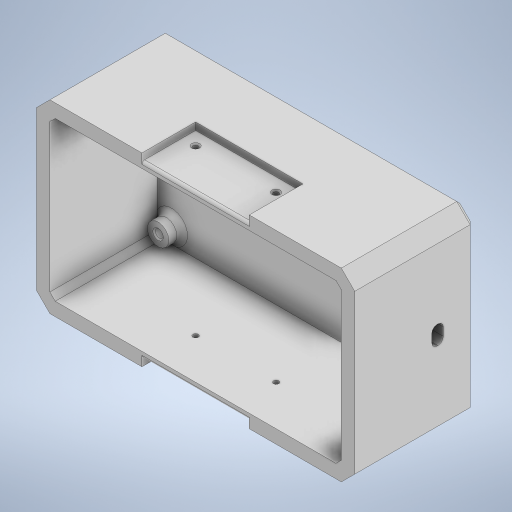
# Autodesk Inventor part: 컨버터 하우징
Saved by Autodesk Inventor 2023 (Build 270158000, 158)
## iProperties
Created: 2022-08-19
Part Number: 컨버터 하우징
Material: 일반
Document SubType Name: Modeling
Designer: user
Density: 1 g/cm^3
Appearance: 기본값
Author: user
Autodesk Inventor part; units mm, degrees
ref_plane "YZ Plane" through (0, 0, 0) normal (1, 0, 0) x (0, 1, 0)
ref_plane "XZ Plane" through (0, 0, 0) normal (0, 1, 0) x (-1, 0, 0)
ref_plane "XY Plane" through (0, 0, 0) normal (0, 0, 1) x (1, 0, 0)
sketch "스케치1" plane through (0, 0, 0) normal (0, 0, 1) x (1, 0, 0)
  line L0 (-54.3, -29.5) -> (54.3, -29.5)
  line L1 (54.3, -29.5) -> (54.3, 29.5)
  line L2 (54.3, 29.5) -> (-54.3, 29.5)
  line L3 (-54.3, 29.5) -> (-54.3, -29.5)
  line L4 (-54.3, -29.5) -> (54.3, 29.5) construction
  line L5 (54.3, -29.5) -> (-54.3, 29.5) construction
  circle A0 centre (-49, 23.75) radius 4
  line L6 (-59.3, 34.5) -> (59.3, 34.5)
  line L7 (59.3, 34.5) -> (59.3, -34.5)
  line L8 (59.3, -34.5) -> (-59.3, -34.5)
  line L9 (-59.3, -34.5) -> (-59.3, 34.5)
  line L10 (0, 0) -> (0, 11.6797)
  line L11 (0, 0) -> (27.7611, 0)
  circle A1 centre (49, 23.75) radius 4
  circle A2 centre (-49, -23.75) radius 4
  circle A3 centre (49, -23.75) radius 4
  dimension "d0" = 108.6
  dimension "d1" = 59
  dimension "d2" = 8
  dimension "d3" = 5
  dimension "d4" = 47.5
  dimension "d5" = 98
  constraints: 24 end point, 4 centre point, 4 parallel, 3 perpendicular, 3 symmetric about line, 2 midpoint, 1 horizontal, 1 vertical, 6 other
  measures "d0" distance of L2.end L1.end
  measures "d1" distance of L1.end L0.end
  measures "d2" diameter of A0
  measures "d3" distance between parallel lines of L2 L6
  measures "d4" distance of A2.centre A0.centre
  measures "d5" distance of A1.centre A0.centre
extrude "돌출1" add sketch "스케치1" against normal blind 5 contours L3 L2 L1 L0 | A0 | L6 L7 L8 L9 | A1 | A2 | A3
extrude "돌출2" add sketch "스케치1" along normal blind 40 contours L6 L7 L8 L9
extrude "돌출4" add sketch "스케치1" along normal blind 5 contours A0 | A1 | A2 | A3
sketch "스케치2" plane through (-49, 23.75, 5) normal (0, 0, 1) x (1, 0, 0)
  circle A0 centre (0, 0) radius 4 projected
  circle A1 centre (98, 0) radius 4 projected
  circle A2 centre (0, -47.5) radius 4 projected
  circle A3 centre (98, -47.5) radius 4 projected
  point P0 (49, -23.75)
hole "구멍1" at (-49, 23.75, 5) at (49, 23.75, 5) at (-49, -23.75, 5) at (49, -23.75, 5) direction (0, 0, -1) diameter 3 depth 9 tip angle 118 countersink diameter 4 countersink angle 90
fillet "모깎기2" radius 2 4 edges at (-53, 23.75, 0) (45, 23.75, 0) (-53, -23.75, 0) (45, -23.75, 0)
ref_plane "작업 평면1" through (0, 0, 7) normal (0, 0, 1) x (1, 0, 0)
sketch "스케치3" plane through (0, 0, 7) normal (0, 0, 1) x (1, 0, 0)
  line L0 (-54.3, 20.9375) -> (-54.3, -20.9375) projected
  line L1 (-59.3, -34.5) -> (-59.3, 34.5) projected
  line L2 (54.3, -20.9375) -> (54.3, 20.9375) projected
  line L3 (59.3, 34.5) -> (59.3, -34.5) projected
  line L4 (-59.3, -1.5) -> (-54.3, -1.5)
  line L5 (-54.3, -1.5) -> (-54.3, 1.5)
  line L6 (-54.3, 1.5) -> (-59.3, 1.5)
  line L7 (-59.3, 1.5) -> (-59.3, -1.5)
  line L8 (-59.3, -1.5) -> (-54.3, 1.5) construction
  line L9 (-54.3, -1.5) -> (-59.3, 1.5) construction
  line L10 (54.3, 3.5) -> (59.3, 3.5)
  line L11 (59.3, 3.5) -> (59.3, -3.5)
  line L12 (59.3, -3.5) -> (54.3, -3.5)
  line L13 (54.3, -3.5) -> (54.3, 3.5)
  line L14 (54.3, 3.5) -> (59.3, -3.5) construction
  line L15 (59.3, 3.5) -> (54.3, -3.5) construction
  point P0 (0, 0)
  point P1 (-59.3, -32.5)
  point P2 (-59.3, 32.5)
  point P3 (59.3, 32.5)
  point P4 (59.3, -32.5)
  point P5 (-56.8, 0)
  point P6 (-56.8, -1.5)
  point P7 (56.8, 0)
  point P8 (59.3, 3.5)
  point P9 (-59.3, -1.5)
  dimension "d24" = 3
  dimension "d25" = 7
  constraints: 24 end point, 5 midpoint, 4 parallel, 4 point on line, 2 horizontal, 2 horizontal alignment, 2 perpendicular
  measures "d24" distance from line of point (-56.8, -1.5) L6
  measures "d25" distance between parallel lines of L12 L10
extrude "돌출5" cut sketch "스케치3" along normal blind 4.3 contours L2 L10 L3 L12
extrude "돌출6" cut sketch "스케치3" along normal blind 2 contours L0 L4 L1 L6
fillet "모깎기4" radius 2 4 edges at (56.8, 3.5, 11.3) (56.8, 3.5, 7) (56.8, -3.5, 11.3) (56.8, -3.5, 7)
fillet "모깎기6" radius 1 4 edges at (-56.8, 1.5, 9) (-56.8, 1.5, 7) (-56.8, -1.5, 7) (-56.8, -1.5, 9)
sketch "스케치4" plane through (0, 0, 40) normal (0, 0, 1) x (1, 0, 0)
  line L0 (-20, 31.8) -> (20, 31.8)
  line L1 (20, 31.8) -> (20, 37.2)
  line L2 (20, 37.2) -> (-20, 37.2)
  line L3 (-20, 37.2) -> (-20, 31.8)
  line L4 (-59.3, 34.5) -> (59.3, 34.5) projected
  line L5 (-20, 31.8) -> (20, 37.2) construction
  line L6 (20, 31.8) -> (-20, 37.2) construction
  line L7 (0, 0) -> (17.5929, 0)
  line L8 (-20, -31.8) -> (20, -31.8)
  line L9 (20, -31.8) -> (20, -37.2)
  line L10 (20, -37.2) -> (-20, -37.2)
  line L11 (-20, -37.2) -> (-20, -31.8)
  line L12 (-20, -31.8) -> (20, -37.2) construction
  line L13 (20, -31.8) -> (-20, -37.2) construction
  line L14 (-59.3, -34.5) -> (59.3, -34.5) projected
  point P0 (0, 34.5)
  point P1 (-57.3, 34.5)
  point P2 (57.3, 34.5)
  point P3 (0, -34.5)
  point P4 (-57.3, -34.5)
  point P5 (57.3, -34.5)
  dimension "d34" = 40
  dimension "d35" = 5.4
  constraints: 26 end point, 5 symmetric about line, 3 midpoint, 2 horizontal, 2 parallel, 1 perpendicular
  measures "d34" distance of L2.end L1.end
  measures "d35" distance of L1.end L0.end
extrude "돌출7" cut sketch "스케치4" against normal blind 20
sketch "스케치5" plane through (-20, -31.8, 40) normal (0, -1, 0) x (1, 0, 0)
  circle A0 centre (5, -15) radius 1
  line L0 (74.3, 0) -> (-34.3, 0) projected
  line L1 (20, 0) -> (20, -11.6914)
  circle A1 centre (35, -15) radius 1
  point P0 (20, -40)
  dimension "d38" = 2
  dimension "d39" = 15
  dimension "d40" = 15
  constraints: 2 centre point, 2 end point, 1 midpoint, 1 symmetric about line, 1 vertical, 1 other
  measures "d38" diameter of A0
  measures "d39" distance from line of L1 A0.centre
  measures "d40" distance from line of L0 A0.centre
extrude "돌출8" cut sketch "스케치5" against normal up to surface (63.6 mm away)
chamfer "모따기1" distance 0.5 angle 45 4 edges at (-16, -31.8, 25) (14, -31.8, 25) (-16, 31.8, 25) (14, 31.8, 25)
chamfer "모따기2" distance 5 angle 45 4 edges at (-59.3, 34.5, 17.5) (-59.3, -34.5, 17.5) (59.3, -34.5, 17.5) (59.3, 34.5, 17.5)
chamfer "모따기3" distance 2 angle 45 4 edges at (-54.3, 29.5, 20) (54.3, 29.5, 20) (54.3, -29.5, 20) (-54.3, -29.5, 20)
fillet "모깎기7" radius 1 2 edges at (0, -31.8, 40) (0, 31.8, 40)
chamfer "모따기4" distance 2 angle 45 8 edges at (-56.8, -32, -5) (-59.3, 0, -5) (0, -34.5, -5) (0, 34.5, -5) (-56.8, 32, -5) (59.3, 0, -5) (56.8, -32, -5) (56.8, 32, -5)
